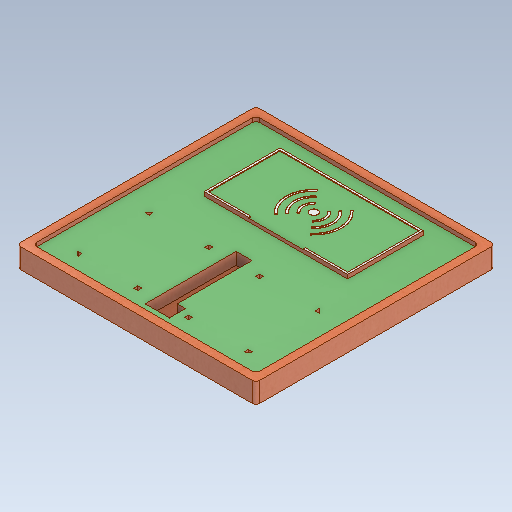
# Autodesk Inventor part: Board
Saved by Autodesk Inventor 2021 (Build 250183000, 183)
## iProperties
Created: 2021-03-16
Part Number: Board
Material: Generic
Document SubType Name: Modeling
Designer: calst
Density: 1 g/cm^3
Appearance: Walnut - Natural Polished
Author: calst
Autodesk Inventor part; units mm, degrees
ref_plane "YZ Plane" through (0, 0, 0) normal (1, 0, 0) x (0, 1, 0)
ref_plane "XZ Plane" through (0, 0, 0) normal (0, 1, 0) x (-1, 0, 0)
ref_plane "XY Plane" through (0, 0, 0) normal (0, 0, 1) x (1, 0, 0)
sketch "Sketch1" plane through (0, 0, 0) normal (0, 1, 0) x (-1, 0, 0)
  line L0 (0, 0) -> (300, 0)
  line L1 (300, 0) -> (300, -300)
  line L2 (300, -300) -> (0, -300)
  line L3 (0, -300) -> (0, 0)
  dimension "d0" = 300
  dimension "d1" = 300
  constraints: 8 end point, 2 parallel, 1 horizontal, 1 perpendicular
  measures "d0" distance of L0.end L1.end
  measures "d1" distance of L0.start L0.end
extrude "Extrusion1" add sketch "Sketch1" along normal blind 25
sketch "Sketch2" plane through (0, 25, 0) normal (0, 1, 0) x (1, 0, 0)
  line L0 (-290, 290) -> (-10, 290)
  line L1 (-10, 290) -> (-10, 10)
  line L2 (-10, 10) -> (-290, 10)
  line L3 (-290, 10) -> (-290, 290)
  line L4 (-300, 300) -> (-300, 0) projected
  line L5 (0, 300) -> (-300, 300) projected
  line L6 (0, 0) -> (0, 300) projected
  line L7 (-300, 0) -> (0, 0) projected
  dimension "d4" = 10
  dimension "d5" = 10
  dimension "d6" = 10
  dimension "d7" = 10
  constraints: 8 end point, 2 parallel, 1 horizontal, 1 perpendicular
  measures "d4" distance between parallel lines of L4 L3
  measures "d5" distance between parallel lines of L5 L0
  measures "d6" distance between parallel lines of L6 L1
  measures "d7" distance between parallel lines of L7 L2
extrude "Extrusion2" cut sketch "Sketch2" against normal blind 5 contours L0 L1 L2 L3
fillet "Fillet1" radius 5 4 edges at (-300, 12.5, 0) (0, 12.5, 0) (0, 12.5, -300) (-300, 12.5, -300)
fillet "Fillet2" radius 5 4 edges at (-290, 22.5, -290) (-10, 22.5, -290) (-10, 22.5, -10) (-290, 22.5, -10)
sketch "Sketch3" plane through (0, 20, 0) normal (0, 1, 0) x (1, 0, 0)
  line L0 (-240, 270) -> (-60, 270)
  line L1 (-60, 270) -> (-60, 175)
  line L2 (-60, 175) -> (-240, 175)
  line L3 (-240, 175) -> (-240, 270)
  line L4 (-285, 290) -> (-15, 290) projected
  line L5 (-290, 15) -> (-290, 285) projected
  line L6 (-10, 285) -> (-10, 15) projected
  point P0 (0, 0)
  dimension "d12" = 95
  dimension "d13" = 20
  dimension "d14" = 50
  dimension "d15" = 50
  constraints: 8 end point, 2 parallel, 1 horizontal, 1 perpendicular
  measures "d12" distance of L2.end L0.start
  measures "d13" distance between parallel lines of L4 L0
  measures "d14" distance between parallel lines of L5 L3
  measures "d15" distance between parallel lines of L6 L1
extrude "Extrusion3" add sketch "Sketch3" along normal blind 5
sketch "Sketch4" plane through (0, 25, 0) normal (0, 1, 0) x (1, 0, 0)
  line L0 (-237.5, 267.5) -> (-62.5, 267.5)
  line L1 (-62.5, 267.5) -> (-62.5, 177.5)
  line L2 (-62.5, 177.5) -> (-237.5, 177.5)
  line L3 (-237.5, 177.5) -> (-237.5, 267.5)
  line L4 (-60, 270) -> (-240, 270) projected
  line L5 (-240, 270) -> (-240, 175) projected
  line L6 (-240, 175) -> (-60, 175) projected
  line L7 (-60, 175) -> (-60, 270) projected
  line L8 (-184.5, 174.1716) -> (-115.5, 174.1716)
  line L9 (-115.5, 174.1716) -> (-115.5, 180.8284)
  line L10 (-115.5, 180.8284) -> (-184.5, 180.8284)
  line L11 (-184.5, 180.8284) -> (-184.5, 174.1716)
  line L12 (-184.5, 174.1716) -> (-115.5, 180.8284) construction
  line L13 (-115.5, 174.1716) -> (-184.5, 180.8284) construction
  point P0 (0, 0)
  point P1 (-150, 177.5)
  dimension "d18" = 2.5
  dimension "d19" = 2.5
  dimension "d20" = 2.5
  dimension "d21" = 2.5
  dimension "d64" = 69
  constraints: 20 end point, 4 parallel, 3 midpoint, 2 horizontal, 2 perpendicular
  measures "d18" distance between parallel lines of L4 L0
  measures "d19" distance between parallel lines of L5 L3
  measures "d20" distance between parallel lines of L6 L2
  measures "d21" distance between parallel lines of L7 L1
  measures "d64" distance of L10.end L9.end
extrude "Extrusion4" cut sketch "Sketch4" against normal blind 1 contours L0 L1 L2 L9 L10 L11 L3 | L11 L10 L9 L2
sketch "Sketch5" plane through (0, 24, 0) normal (0, 1, 0) x (1, 0, 0)
  line L0 (-237.5, 177.5) -> (-237.5, 267.5) projected
  line L1 (-62.5, 267.5) -> (-62.5, 177.5) projected
  circle A0 centre (-150.0001, 222.5) radius 5
  line L2 (-129.1072, 197.6055) -> (-127.5001, 195.6905)
  arc A1 (-140.3572, 211.0103) -> (-140.3575, 233.99) centre (-150.0001, 222.5) ccw
  arc A2 (-159.6427, 233.99) -> (-159.6429, 211.0103) centre (-150.0001, 222.5) ccw
  arc A3 (-141.9644, 212.9252) -> (-141.9646, 232.075) centre (-150.0001, 222.5) ccw
  arc A4 (-158.0356, 232.075) -> (-158.0358, 212.9252) centre (-150.0001, 222.5) ccw
  arc A5 (-135.5358, 205.2654) -> (-135.5362, 239.735) centre (-150.0001, 222.5) ccw
  arc A6 (-164.464, 239.735) -> (-164.4644, 205.2654) centre (-150.0001, 222.5) ccw
  arc A7 (-133.9286, 203.3504) -> (-133.9291, 241.65) centre (-150.0001, 222.5) ccw
  arc A8 (-166.0711, 241.65) -> (-166.0715, 203.3504) centre (-150.0001, 222.5) ccw
  arc A9 (-129.1072, 197.6055) -> (-129.1078, 247.395) centre (-150.0001, 222.5) ccw
  arc A10 (-170.8924, 247.395) -> (-170.8929, 197.6055) centre (-150.0001, 222.5) ccw
  arc A11 (-127.5001, 195.6905) -> (-127.5007, 249.31) centre (-150.0001, 222.5) ccw
  arc A12 (-172.4995, 249.31) -> (-172.5001, 195.6905) centre (-150.0001, 222.5) ccw
  line L3 (-129.1078, 247.395) -> (-127.5007, 249.31)
  line L4 (-141.9646, 232.075) -> (-140.3575, 233.99)
  line L5 (-135.5362, 239.735) -> (-133.9291, 241.65)
  line L6 (-135.5358, 205.2654) -> (-133.9286, 203.3504)
  line L7 (-141.9644, 212.9252) -> (-140.3572, 211.0103)
  line L8 (-158.0356, 232.075) -> (-159.6427, 233.99)
  line L9 (-164.464, 239.735) -> (-166.0711, 241.65)
  line L10 (-170.8924, 247.395) -> (-172.4995, 249.31)
  line L11 (-158.0358, 212.9252) -> (-159.6429, 211.0103)
  line L12 (-164.4644, 205.2654) -> (-166.0715, 203.3504)
  line L13 (-170.8929, 197.6055) -> (-172.5001, 195.6905)
  line L14 (-237.5, 222.5) -> (-62.5, 222.5)
  line L15 (-62.5, 267.5) -> (-62.5, 177.5) projected
  line L16 (-240, 175) -> (-60, 175) projected
  line L17 (-150, 175) -> (-150, 270)
  line L18 (-240, 270) -> (-60, 270) projected
  point P0 (0, 0)
  dimension "d53" = 10
  constraints: 28 end point, 24 point on circle, 13 centre point, 6 coincident, 4 midpoint
  measures "d53" diameter of A0
extrude "Extrusion6" cut sketch "Sketch5" against normal blind 0.5
sketch "Sketch8" plane through (0, 25, 0) normal (0, 1, 0) x (1, 0, 0)
  line L0 (-240, 175) -> (-240, 270) projected
  line L1 (-240, 175) -> (-150, 175)
  line L2 (-240, 175) -> (-60, 175) projected
  line L3 (-150, 175) -> (-184.25, 175)
  line L4 (-184.25, 175) -> (-184.25, 177.5)
  line L5 (-62.5, 177.5) -> (-237.5, 177.5) projected
  line L6 (-187.5, 180) -> (-112.5, 180) projected
  line L7 (-150, 175) -> (-115.75, 175)
  line L8 (-115.75, 175) -> (-115.75, 177.5)
  line L9 (-184.25, 177.5) -> (-115.75, 177.5)
  point P0 (0, 0)
  dimension "d72" = 34.25
  dimension "d74" = 34.25
  constraints: 12 end point, 4 point on line, 2 perpendicular, 1 collinear, 1 midpoint
  measures "d72" distance of L1.end L3.end
  measures "d74" distance of L1.end L7.end
extrude "Extrusion9" cut sketch "Sketch8" against normal blind 1
sketch "Sketch11" plane through (0, 0, 0) normal (0, -1, 0) x (1, 0, 0)
  line L0 (-135.0001, -207.625) -> (-135.0001, -222.5) projected
  line L1 (-165.0001, -267.125) -> (-165.0001, -240.3738) projected
  line L2 (-135.0001, -207.625) -> (-165.0001, -207.625)
  line L3 (-165.0001, -207.625) -> (-165.0001, -267.125)
  line L4 (-165.0001, -267.125) -> (-135.0001, -267.125)
  line L5 (-135.0001, -267.125) -> (-135.0001, -207.625)
  point P0 (0, 0)
  constraints: 8 end point, 2 parallel, 1 horizontal, 1 perpendicular
extrude "Extrusion11" cut sketch "Sketch11" against normal blind 6
sketch "Sketch12" plane through (0, 20, 0) normal (0, 1, 0) x (1, 0, 0)
  line L0 (-184.25, 175) -> (-184.25, 177.5) projected
  line L1 (-60, 175) -> (-240, 175) projected
  line L2 (-184.25, 31) -> (-179.25, 31)
  line L3 (-179.25, 31) -> (-179.25, 36)
  line L4 (-179.25, 36) -> (-184.25, 36)
  line L5 (-184.25, 36) -> (-184.25, 31)
  line L6 (-115.75, 31) -> (-120.75, 31)
  line L7 (-120.75, 31) -> (-120.75, 36)
  line L8 (-120.75, 36) -> (-115.75, 36)
  line L9 (-115.75, 36) -> (-115.75, 31)
  line L10 (-115.75, 125) -> (-120.75, 125)
  line L11 (-120.75, 125) -> (-120.75, 120)
  line L12 (-120.75, 120) -> (-115.75, 120)
  line L13 (-115.75, 120) -> (-115.75, 125)
  line L14 (-184.25, 125) -> (-179.25, 125)
  line L15 (-179.25, 125) -> (-179.25, 120)
  line L16 (-179.25, 120) -> (-184.25, 120)
  line L17 (-184.25, 120) -> (-184.25, 125)
  line L18 (-160, 120) -> (-160, 31)
  line L19 (-140, 41) -> (-140, 125)
  line L20 (-160, 125) -> (-160, 120)
  line L21 (-160, 125) -> (-160, 135)
  line L22 (-160, 135) -> (-140, 135)
  line L23 (-140, 135) -> (-140, 125)
  line L24 (-160, 31) -> (-160, 21)
  line L25 (-160, 21) -> (-140, 21)
  line L26 (-129.545, 41) -> (-129.545, 21)
  line L27 (-129.545, 21) -> (-140, 21)
  line L28 (-129.545, 41) -> (-140, 41)
  point P0 (0, 0)
  dimension "d87" = 50
  dimension "d90" = 94
  dimension "d91" = 5
  dimension "d92" = 5
  dimension "d93" = 5
  dimension "d100" = 10
  dimension "d101" = 10
  constraints: 54 end point, 9 perpendicular, 8 parallel, 5 point on line, 4 horizontal, 2 vertical
  measures "d87" distance of L0.start L14.start
  measures "d90" distance of L14.start L2.start
  measures "d91" distance of L15.end L16.end
  measures "d92" distance of L14.end L15.end
  measures "d93" distance of L11.end L12.end
  measures "d100" distance of L20.start L21.end
  measures "d101" distance of L18.end L24.end
extrude "Extrusion12" cut sketch "Sketch12" against normal blind 15
sketch "Sketch13" plane through (0, 20, 0) normal (0, 1, 0) x (1, 0, 0)
  line L0 (-120.75, 125) -> (-115.75, 125) projected
  line L1 (-45.75, 125) -> (-40.75, 125)
  line L2 (-40.75, 125) -> (-40.75, 120)
  line L3 (-40.75, 120) -> (-45.75, 120)
  line L4 (-45.75, 120) -> (-45.75, 125)
  line L5 (-45.75, 31.0976) -> (-40.75, 31.0976)
  line L6 (-40.75, 31.0976) -> (-40.75, 36.0976)
  line L7 (-40.75, 36.0976) -> (-45.75, 36.0976)
  line L8 (-45.75, 36.0976) -> (-45.75, 31.0976)
  line L9 (-184.25, 120) -> (-184.25, 125) projected
  line L10 (-254.25, 125) -> (-254.25, 120)
  line L11 (-254.25, 120) -> (-259.25, 120)
  line L12 (-259.25, 120) -> (-259.25, 125)
  line L13 (-259.25, 125) -> (-254.25, 125)
  line L14 (-184.25, 36) -> (-179.25, 36) projected
  line L15 (-254.25, 36) -> (-254.25, 31)
  line L16 (-254.25, 31) -> (-259.25, 31)
  line L17 (-259.25, 31) -> (-259.25, 36)
  line L18 (-259.25, 36) -> (-254.25, 36)
  point P0 (0, 0)
  dimension "d105" = 70
  dimension "d106" = 5
  dimension "d107" = 5
  dimension "d108" = 5
  dimension "d109" = 5
  dimension "d110" = 70
  dimension "d111" = 5
  dimension "d112" = 70
  dimension "d113" = 5
  constraints: 32 end point, 8 perpendicular, 4 parallel, 2 horizontal
  measures "d105" distance of L0.end L1.start
  measures "d106" distance of L2.end L3.end
  measures "d107" distance of L1.end L2.end
  measures "d108" distance of L7.end L6.end
  measures "d109" distance of L5.end L6.end
  measures "d110" distance of L9.end L10.start
  measures "d111" distance of L10.end L11.end
  measures "d112" distance of L14.start L15.start
  measures "d113" distance of L15.start L15.end
extrude "Extrusion13" cut sketch "Sketch13" against normal blind 15
chamfer "Chamfer1" distance 4 angle 45 2 edges at (-259.25, 12.5, -125) (-40.75, 12.5, -125)
chamfer "Chamfer2" distance 4 angle 45 2 edges at (-40.75, 12.5, -31.0976) (-259.25, 12.5, -31)
body "Solid1"
